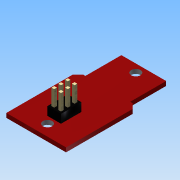
# Autodesk Inventor part: wheel_encoder
Saved by Autodesk Inventor 2015 (Build 190159000, 159)
## iProperties
Created: 2014-12-09
Part Number: wheel_encoder
Material: Generic
Document SubType Name: Modeling
Designer: Daniel
Density: 1 g/cm^3
Appearance: Default
Author: Daniel
Autodesk Inventor part; units mm, degrees
ref_plane "YZ Plane" through (0, 0, 0) normal (1, 0, 0) x (0, 1, 0)
ref_plane "XZ Plane" through (0, 0, 0) normal (0, 1, 0) x (-1, 0, 0)
ref_plane "XY Plane" through (0, 0, 0) normal (0, 0, 1) x (1, 0, 0)
sketch "Sketch1" plane through (0, 0, 0) normal (0, 1, 0) x (-1, 0, 0)
  line L0 (11.176, 13.3985) -> (-11.176, 13.3985)
  line L1 (-11.176, 13.3985) -> (-11.176, -11.4935)
  line L2 (11.176, -11.4935) -> (11.176, 13.3985)
  line L3 (11.176, 13.3985) -> (-11.176, -13.3985) construction
  line L4 (0, 20.6375) -> (0, -33.0464)
  line L5 (-8.382, -13.3985) -> (-8.382, -26.8605)
  line L6 (-8.382, -26.8605) -> (8.382, -26.8605)
  line L7 (8.382, -26.8605) -> (8.382, -13.3985)
  line L8 (9.271, -13.3985) -> (11.176, -11.4935)
  line L9 (-9.271, -13.3985) -> (-11.176, -11.4935)
  line L10 (-9.271, -13.3985) -> (-8.382, -13.3985)
  line L11 (8.382, -13.3985) -> (9.271, -13.3985)
  point P0 (0, 0)
  point P1 (11.176, -13.3985)
  point P2 (0, 0)
  dimension "d0" = 22.352
  dimension "d1" = 26.797
  dimension "d2" = 16.764
  dimension "d3" = 13.462
  dimension "d4" = 1.905
  dimension "d5" = 1.905
  dimension "d6" = 1.905
  dimension "d7" = 1.905
  constraints: 24 end point, 4 parallel, 3 point on line, 1 coincident, 1 horizontal, 1 midpoint, 1 perpendicular, 1 vertical
  measures "d0" diameter of L2 L4
  measures "d1" distance of point (11.176, -13.398) L0.start
  measures "d2" distance of L6.end L5.end
  measures "d3" distance of L5.start L5.end
  measures "d4" distance of L8.start point (11.176, -13.398)
  measures "d5" distance of L2.start point (11.176, -13.398)
  measures "d6" distance of L9.start L3.end
  measures "d7" distance of L1.end L3.end
extrude "Extrusion1" add sketch "Sketch1" along normal blind 1.6002
sketch "Sketch2" plane through (0, 1.6002, 0) normal (0, 1, 0) x (1, 0, 0)
  line L0 (-11.176, -13.3985) -> (11.176, -13.3985) projected
  line L1 (8.382, 26.8605) -> (-8.382, 26.8605) projected
  line L2 (0, -15.1574) -> (0, 42.0562)
  line L3 (0, -15.1574) -> (57.2136, -15.1574) construction
  point P0 (0, 0)
  point P1 (0, -9.1567)
  point P2 (0, 23.8887)
  dimension "d10" = 4.2418
  dimension "d11" = 2.9718
  dimension "d12" = 90
  constraints: 4 end point, 3 point on line, 1 horizontal, 1 perpendicular
  measures "d10" distance from line of point (0, -9.157) L0
  measures "d11" distance from line of L1 point (0, 23.889)
  measures "d12" angle of L3 L2
hole "Hole1" at (0, 1.6002, 9.1567) at (0, 1.6002, -23.8887) direction (0, -1, 0) diameter 3.4544 end through all clearance for "Flat Head Machine Screw (82)" size "#5" standard "Ansi Unified Screw Threads"
sketch "Sketch3" plane through (0, 1.6002, 0) normal (0, 1, 0) x (1, 0, 0)
  line L0 (-2.54, 0.9525) -> (2.54, 0.9525)
  line L1 (2.54, 0.9525) -> (2.54, -6.6675)
  line L2 (2.54, -6.6675) -> (-2.54, -6.6675)
  line L3 (-2.54, -6.6675) -> (-2.54, 0.9525)
  line L4 (0, 0) -> (0, 29.7759)
  line L5 (0, 0) -> (29.7759, 0) construction
  line L6 (0, 0) -> (0, -24.9457)
  line L7 (0, 0) -> (24.9457, 0) construction
  line L8 (-2.54, 0.9525) -> (2.54, -6.6675) construction
  line L9 (-11.176, -13.3985) -> (11.176, -13.3985) construction
  point P0 (0, -2.8575)
  dimension "d20" = 90
  dimension "d21" = 90
  dimension "d22" = 10.541
  dimension "d23" = 5.08
  dimension "d24" = 7.62
  constraints: 18 end point, 3 horizontal, 3 perpendicular, 2 parallel, 1 midpoint, 1 point on line
  measures "d20" angle of L5 L4
  measures "d21" angle of L6 L7
  measures "d22" distance from line of L9 point (0, -2.857)
  measures "d23" diameter of L2.end L6
  measures "d24" distance between parallel lines of L0 L2
extrude "Extrusion2" add sketch "Sketch3" along normal blind 3.175
sketch "Sketch4" plane through (0, 4.7752, 0) normal (0, 1, 0) x (1, 0, 0)
  line L0 (0, 1.9235) -> (0, -7.9336)
  line L1 (-5.0807, -2.8575) -> (5.7317, -2.8575)
  line L2 (2.54, 0.9525) -> (-2.54, 0.9525) projected
  line L3 (2.54, -6.6675) -> (2.54, 0.9525) projected
  line L4 (-1.778, 0.1905) -> (-0.762, 0.1905)
  line L5 (-0.762, 0.1905) -> (-0.762, -0.8255)
  line L6 (-0.762, -0.8255) -> (-1.778, -0.8255)
  line L7 (-1.778, -0.8255) -> (-1.778, 0.1905)
  point P0 (0, 0)
  point P1 (0, 0.9525)
  point P2 (2.54, -2.8575)
  dimension "d27" = 1.016
  dimension "d28" = 1.016
  dimension "d29" = 1.524
  dimension "d30" = 4.064
  constraints: 12 end point, 2 horizontal, 2 midpoint, 2 parallel, 2 point on line, 1 perpendicular, 1 vertical
  measures "d27" distance of L5.end L6.end
  measures "d28" distance of L4.end L5.end
  measures "d29" diameter of L5 L0
  measures "d30" diameter of L6 L1
extrude "Extrusion3" add sketch "Sketch4" along normal blind 5.9944 contours L4 L5 L6 L7
pattern_linear "Rectangular Pattern1" count 2 spacing 2.54 along (1, 0, 0) count 3 spacing 2.54 along (0, 0, 1) of "Extrusion3"
sketch "Sketch5" plane through (0, 0, 0) normal (0, -1, 0) x (1, 0, 0)
  line L0 (0, 15.1213) -> (0, -35.4386)
  line L1 (6.985, -1.5875) -> (4.318, -1.5875)
  line L2 (4.318, -1.5875) -> (4.318, -4.9403)
  line L3 (4.318, -4.9403) -> (6.985, -4.9403)
  line L4 (6.985, -4.9403) -> (6.985, -1.5875)
  line L5 (-11.176, 13.3985) -> (11.176, 13.3985) projected
  line L6 (-4.318, -4.9403) -> (-6.985, -4.9403)
  line L7 (-6.985, -4.9403) -> (-6.985, -1.5875)
  line L8 (-6.985, -1.5875) -> (-4.318, -1.5875)
  line L9 (-4.318, -1.5875) -> (-4.318, -4.9403)
  point P0 (0, 0)
  dimension "d39" = 2.667
  dimension "d40" = 3.3528
  dimension "d41" = 8.636
  dimension "d42" = 14.986
  dimension "d43" = 8.636
  constraints: 18 end point, 4 parallel, 2 equal length, 2 horizontal, 2 perpendicular, 1 collinear, 1 point on line, 1 vertical
  measures "d39" distance of L3.end L2.end
  measures "d40" distance of L2.end L1.end
  measures "d41" diameter of L2 L0
  measures "d42" distance between parallel lines of L1 L5
  measures "d43" diameter of L9 L0
extrude "Extrusion4" add sketch "Sketch5" along normal blind 1.651
equation "\"d5\" = d4"
equation "\"d6\" = d4"
equation "\"d7\" = d6"
equation "\"d43\" = d41"
body "Solid1"
